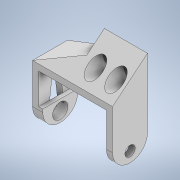
# Autodesk Inventor part: juncao7
Saved by Autodesk Inventor 2022.2 (Build 262287010, 287A)
## iProperties
Created: 2021-08-04
Part Number: juncao7
Material: Generic
Document SubType Name: Modeling
Designer: nakai
Density: 1 g/cm^3
Appearance: Default
Author: nakai
Autodesk Inventor part; units mm, degrees
ref_plane "YZ Plane" through (0, 0, 0) normal (1, 0, 0) x (0, 1, 0)
ref_plane "XZ Plane" through (0, 0, 0) normal (0, 1, 0) x (-1, 0, 0)
ref_plane "XY Plane" through (0, 0, 0) normal (0, 0, 1) x (1, 0, 0)
sketch "Sketch1" plane through (0, 0, 0) normal (0, 0, 1) x (1, 0, 0)
  line L0 (0, 0) -> (5, 0)
  line L1 (5, 0) -> (5, 25)
  line L2 (5, 25) -> (0, 25)
  line L3 (0, 25) -> (0, 0)
  line L4 (36, 25) -> (39, 25)
  line L5 (39, 25) -> (39, 0)
  line L6 (39, 0) -> (36, 0)
  line L7 (36, 0) -> (36, 25)
  line L8 (0, 25) -> (39, 25)
  line L9 (39, 25) -> (39, 42)
  line L10 (39, 42) -> (0, 42)
  line L11 (0, 42) -> (0, 25)
  line L12 (5, 25) -> (3, 25)
  line L13 (3, 25) -> (3, 10)
  line L14 (3, 10) -> (5, 10)
  line L15 (5, 10) -> (5, 25)
  dimension "d0" = 5
  dimension "d1" = 25
  dimension "d2" = 3
  dimension "d3" = 25
  dimension "d4" = 31
  dimension "d6" = 17
  dimension "d48" = 0
  dimension "d54" = 2
  dimension "d55" = 15
  constraints: 32 end point, 8 parallel, 4 horizontal, 4 perpendicular, 1 point on line
  measures "d0" distance of L2.end L1.end
  measures "d1" distance of L1.end L0.end
  measures "d2" distance of L5.end L6.end
  measures "d3" distance of L4.end L5.end
  measures "d4" distance between parallel lines of L7 L1
  measures "d6" distance of L9.end L8.end
  measures "d48" distance between parallel lines of L9 L5
  measures "d54" distance of L14.end L13.end
  measures "d55" distance of L13.end L12.end
extrude "Extrusion1" add sketch "Sketch1" along normal blind 17 contours L3 L2 L13 L14 L1 L0 | L11 L10 L9 L4 L8 L2 | L4 L5 L6 L7
sketch "Sketch2" plane through (39, 0, 0) normal (1, 0, 0) x (0, 0, -1)
  line L0 (-17, 28) -> (-17, 42)
  line L1 (0, 42) -> (-17, 42) projected
  line L2 (-17, 42) -> (0, 42)
  line L3 (0, 42) -> (-17, 28)
  point P0 (0, 0)
  dimension "d9" = 14
  constraints: 6 end point, 1 perpendicular
  measures "d9" distance of L0.start L0.end
extrude "Extrusion2" cut sketch "Sketch2" against normal up to surface (39 mm away)
sketch "Sketch3" plane through (0, 0, 0) normal (0, 0, -1) x (-1, 0, 0)
  line L0 (0, 42) -> (0, 0) projected
  line L1 (0, 42) -> (-15, 42)
  line L2 (-15, 42) -> (-15, 29)
  line L3 (-15, 29) -> (0, 29)
  line L4 (0, 29) -> (0, 42)
  point P0 (0, 29)
  dimension "d12" = 15
  dimension "d13" = 13
  constraints: 8 end point, 2 parallel, 1 horizontal, 1 perpendicular
  measures "d12" distance of L3.end L2.end
  measures "d13" distance of L2.end L1.end
extrude "Extrusion3" cut sketch "Sketch3" against normal up to surface (17 mm away)
sketch "Sketch4" plane through (0, 0, 17) normal (0, 0, 1) x (1, 0, 0)
  line L0 (39, 0) -> (39, 42) projected
  line L1 (39, 42) -> (19, 42)
  line L2 (19, 42) -> (19, 25)
  line L3 (19, 25) -> (39, 25)
  line L4 (39, 25) -> (39, 42)
  circle A0 centre (34, 33.5) radius 3.5
  circle A1 centre (24, 33.5) radius 3.5
  point P0 (0, 0)
  dimension "d16" = 20
  dimension "d17" = 17
  dimension "d18" = 7
  dimension "d19" = 7
  dimension "d20" = 8.5
  dimension "d21" = 5
  dimension "d22" = 8.5
  dimension "d23" = 5
  constraints: 8 end point, 2 centre point, 2 parallel, 1 horizontal, 1 perpendicular
  measures "d16" distance of L0.end L1.end
  measures "d17" distance of L1.end L2.end
  measures "d18" diameter of A0
  measures "d19" diameter of A1
  measures "d20" distance from line of L1 A0.centre
  measures "d21" distance from line of L0 A0.centre
  measures "d22" distance from line of L1 A1.centre
  measures "d23" distance from line of L2 A1.centre
extrude "Extrusion4" cut sketch "Sketch4" against normal blind 14 contours A0 | A1
sketch "Sketch5" plane through (0, 0, 3) normal (0, 0, 1) x (1, 0, 0)
  circle A0 centre (34, 33.5) radius 3.5 projected
  circle A1 centre (34, 33.5) radius 1.5
  circle A2 centre (24, 33.5) radius 3.5 projected
  circle A3 centre (24, 33.5) radius 1.5
  point P0 (0, 0)
  point P1 (32.4191, 39.5294)
  point P2 (27.5809, 39.5294)
  point P3 (22.4191, 39.5294)
  point P4 (17.5809, 39.5294)
  dimension "d26" = 3
  dimension "d27" = 3
  constraints: 2 centre point, 2 coincident, 2 other
  measures "d26" diameter of A1
  measures "d27" diameter of A3
extrude "Extrusion5" cut sketch "Sketch5" against normal up to surface (3 mm away) contours A1 | A3
sketch "Sketch6" plane through (15, 29, 0) normal (-1, 0, 0) x (0, 0, 1)
  line L0 (0, 0) -> (15.7857, 0) projected
  line L1 (0, 13) -> (15.7857, 0)
  line L2 (15.7857, 0) -> (0, 0)
  line L3 (0, 0) -> (0, 13)
  line L4 (0, 0) -> (0, 13) projected
  point P0 (0, -29)
  constraints: 6 end point, 2 point on line
extrude "Extrusion6" add sketch "Sketch6" along normal up to surface (15 mm away)
sketch "Sketch7" plane through (0, 0, 17) normal (0, 0, 1) x (1, 0, 0)
  line L0 (39, 28) -> (0, 28) projected
  line L1 (0, 28) -> (18, 28)
  line L2 (18, 28) -> (18, 35)
  line L3 (18, 35) -> (0, 28)
  line L4 (18, 35) -> (18, 42)
  line L5 (0, 28) -> (0, 42) projected
  line L6 (18, 42) -> (0, 42)
  line L7 (0, 42) -> (0, 28)
  point P0 (0, 0)
  dimension "d32" = 18
  dimension "d33" = 7
  dimension "d34" = 7
  constraints: 12 end point, 1 collinear, 1 perpendicular, 1 point on line, 1 vertical
  measures "d32" distance of L0.end L1.end
  measures "d33" distance of L1.end L2.end
  measures "d34" distance of L2.end L4.end
extrude "Extrusion7" cut sketch "Sketch7" against normal up to surface (17 mm away) contours L5 L6 L4 L3
sketch "Sketch8" plane through (0, 0, 0) normal (-1, 0, 0) x (0, 0, 1)
  circle A0 centre (8.5, 5) radius 3.75
  line L0 (0, 0) -> (17, 0) projected
  line L1 (17, 28) -> (17, 0) projected
  dimension "d37" = 7.5
  dimension "d38" = 5
  dimension "d39" = 8.5
  constraints: 1 centre point
  measures "d37" diameter of A0
  measures "d38" distance from line of L0 A0.centre
  measures "d39" distance from line of L1 A0.centre
extrude "Extrusion8" cut sketch "Sketch8" against normal up to surface (5 mm away)
sketch "Sketch9" plane through (39, 0, 17) normal (1, 0, 0) x (0, 0, -1)
  circle A0 centre (8.5, 5) radius 2.5
  line L0 (17, 0) -> (0, 0) projected
  line L1 (0, 0) -> (0, 28) projected
  dimension "d42" = 5
  dimension "d43" = 5
  dimension "d44" = 8.5
  constraints: 1 centre point
  measures "d42" diameter of A0
  measures "d43" distance from line of L0 A0.centre
  measures "d44" distance from line of L1 A0.centre
extrude "Extrusion9" cut sketch "Sketch9" against normal up to surface (3 mm away)
fillet "Fillet1" radius 8.5 4 edges at (2.5, 0, 17) (37.5, 0, 17) (37.5, 0, 0) (2.5, 0, 0)
sketch "Sketch10" plane through (0, 28, 0) normal (-1, 0, 0) x (0, 0, 1)
  circle A0 centre (8.5, -8) radius 2
  circle A1 centre (8.5, -23) radius 3.75
  line L0 (10.4863, -7.7667) -> (12.2244, -22.5625)
  line L1 (6.5137, -7.7667) -> (4.7756, -22.5625)
  circle A2 centre (8.5, -23) radius 3.75 projected
  circle A3 centre (8.5, -23) radius 3.5
  point P0 (0, -28)
  dimension "d49" = 4
  dimension "d50" = 15
  dimension "d51" = 0
  constraints: 4 end point, 4 point on circle, 4 tangent, 3 centre point, 1 coincident
  measures "d49" diameter of A0
  measures "d50" distance of A1.centre A0.centre
  measures "d51" horizontal distance of A1.centre A0.centre
extrude "Extrusion10" cut sketch "Sketch10" against normal blind 3 contours A0 | A0 L0 A1 L1
body "Solid1"
